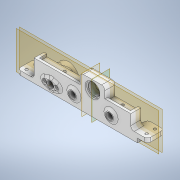
# Autodesk Inventor part: MotorBracket_v6.2
Saved by Autodesk Inventor 2022 (Build 260153000, 153)
## iProperties
Created: 2022-01-31
Part Number: MotorBracket_v6.2
Material: ABS プラスチック
Document SubType Name: Modeling
Designer: shiokaze
Density: 1.06 g/cm^3
Appearance: 滑らか - 白
Mass: 5.74152 g
Surface Area: 41.0545 cm^2
Volume: 5.41653 cm^3
Author: shiokaze
Autodesk Inventor part; units mm, degrees
ref_plane "YZ Plane" through (0, 0, 0) normal (1, 0, 0) x (0, 1, 0)
ref_plane "XZ Plane" through (0, 0, 0) normal (0, 1, 0) x (-1, 0, 0)
ref_plane "XY Plane" through (0, 0, 0) normal (0, 0, 1) x (1, 0, 0)
sketch "スケッチ2" plane through (0, 0, 0) normal (0, 0, 1) x (1, 0, 0)
  line L0 (-46.5, 9.7) -> (31.5, 9.7)
  line L1 (31.5, 9.7) -> (31.5, -9.7)
  line L2 (31.5, -9.7) -> (-46.5, -9.7)
  line L3 (-46.5, -9.7) -> (-46.5, 9.7)
  line L4 (-46.5, 9.7) -> (31.5, -9.7)
  line L5 (31.5, 9.7) -> (-46.5, -9.7)
  line L6 (-46.5, 9.7) -> (-8.95, 9.7)
  line L7 (-8.95, 9.7) -> (-8.95, -7.2)
  line L8 (-8.95, -7.2) -> (-46.5, -7.2)
  line L9 (-46.5, -7.2) -> (-46.5, 9.7)
  line L10 (31.5, 9.7) -> (5.95, 9.7)
  line L11 (5.95, 9.7) -> (5.95, -4.7)
  line L12 (5.95, -4.7) -> (31.5, -4.7)
  line L13 (31.5, -4.7) -> (31.5, 9.7)
  line L14 (-36.448454, -7.2) -> (-36.5, -7.2)
  line L15 (-36.5, -7.2) -> (-36.5, 3.5)
  line L16 (-36.5, 3.5) -> (-8.95, 3.5)
  line L17 (-8.95, 3.5) -> (-8.95, -0.360641)
  line L18 (5.95, -4.7) -> (21.5, -4.7)
  line L19 (21.5, -4.7) -> (21.5, 3.5)
  line L20 (21.5, 3.5) -> (5.95, 3.5)
  line L21 (5.95, 3.5) -> (5.95, -4.7)
  line L22 (31.5, -9.7) -> (25.5, -9.7)
  line L23 (25.5, -9.7) -> (25.5, -7.2)
  line L24 (25.5, -7.2) -> (31.5, -7.2)
  line L25 (31.5, -7.2) -> (31.5, -9.7)
  line L26 (-7.5, 0) -> (0, 0)
  point P0 (-7.5, 0)
  point P1 (5.95, 9.7)
  point P2 (-8.95, 9.7)
  point P3 (-8.95, 3.5)
  point P4 (-36.5, -7.2)
  point P5 (-46.5, -7.2)
  point P6 (31.5, -7.2)
  point P7 (31.5, -4.7)
  point P8 (21.5, -4.7)
  dimension "d0" = 78
  dimension "d1" = 19.4
  dimension "d15" = 37.55
  dimension "d16" = 2.5
  dimension "d17" = 25.55
  dimension "d18" = 6
  dimension "d19" = 2.5
  dimension "d20" = 10
  dimension "d21" = 10
  dimension "d26" = 7.5
  dimension "d188" = 10.7
  dimension "d241" = 5
  constraints: 54 end point, 12 parallel, 7 horizontal, 6 perpendicular, 3 collinear, 2 midpoint, 2 point on line, 1 coincident
  measures "d0" distance of L0.start L0.end
  measures "d1" distance of L0.end L1.end
  measures "d15" distance of L7.end L8.end
  measures "d16" distance between parallel lines of L2 L8
  measures "d17" distance of L12.end L11.end
  measures "d18" distance of L23.end L24.end
  measures "d19" distance of L22.end L23.end
  measures "d20" distance between parallel lines of L1 L19
  measures "d21" distance between parallel lines of L3 L15
  measures "d26" distance of L26.start L26.end
  measures "d188" distance between parallel lines of L16 L8
  measures "d241" distance between parallel lines of L18 L2
extrude "押し出し1" add sketch "スケッチ2" along normal blind 6 contours L0 L11 L5 L4 L7 | L8 L5 L3 | L16 L7 L4 | L4 L7 L5 L8 L15 L16 | L5 L8 L7 L4 L11 L12 L23 L2 | L4 L5 L7 | L20 L5 L11 | L5 L7 L8 | L5 L11 L4 | L1 L24 L23 L4 L12 | L20 L19 L12 L4 L11 L5 | L4 L12 L11
sketch "スケッチ8" plane through (0, 0, 6) normal (0, 0, 1) x (1, 0, 0)
  circle A0 centre (-1.5, 4.258894) radius 3.8 construction
  circle A1 centre (9.625, -3.3) radius 9.65 construction
  circle A2 centre (-12.625, -3.3) radius 9.65 construction
  circle A3 centre (-26.001939, -4.7) radius 3.8 construction
  line L0 (-46.5, -9.7) -> (25.5, -9.7) construction
  circle A4 centre (-12.625, -3.3) radius 10.5
  circle A5 centre (9.625, -3.3) radius 10.5
  line L1 (-2.125, -3.3) -> (-0.875, -3.3)
  line L2 (-12.625, -3.3) -> (-1.5, 4.258894) construction
  line L3 (-1.5, 4.258894) -> (9.625, -3.3) construction
  line L4 (-26.001939, -4.7) -> (-12.625, -3.3) construction
  line L5 (-46.5, -9.7) -> (25.5, -9.7)
  line L6 (-46.5, -9.7) -> (25.5, -9.7)
  line L7 (25.5, -9.7) -> (25.5, -11.3)
  line L8 (25.5, -11.3) -> (-46.5, -11.3) construction
  line L9 (-46.5, -11.3) -> (-46.5, -9.7)
  line L10 (-46.5, -11.3) -> (25.5, -11.3)
  line L11 (25.5, -11.3) -> (25.5, -13.8)
  line L12 (25.5, -13.8) -> (-46.5, -13.8) construction
  line L13 (-46.5, -13.8) -> (-46.5, -11.3)
  line L14 (25.5, -9.7) -> (25.5, -7.2)
  line L15 (5.95, 9.7) -> (-8.95, 9.7)
  circle A6 centre (-26.001939, -4.7) radius 5
  point P0 (0, 0)
  point P1 (-1.5, 9.7)
  dimension "d123" = 21
  dimension "d124" = 21
  dimension "d29" = 7.6
  dimension "d30" = 19.3
  dimension "d31" = 19.3
  dimension "d32" = 7.6
  dimension "d132" = 1.25
  dimension "d147" = 1.6
  dimension "d148" = 2.5
  dimension "d164" = 10
  constraints: 24 end point, 7 coincident, 5 centre point, 4 horizontal, 4 parallel, 2 collinear, 2 equal length, 2 horizontal alignment, 2 perpendicular, 2 point on line, 2 tangent, 1 midpoint, 1 vertical alignment, 4 other
  measures "d29" diameter of A0
  measures "d30" diameter of A2
  measures "d31" diameter of A1
  measures "d32" diameter of A3
  measures "d132" distance of L1.start L1.end
  measures "d147" distance of L6.end L7.end
  measures "d148" distance of L10.end L11.end
  measures "d164" diameter of A6
hole "穴1" at (-12.625, -3.3, 6) at (9.625, -3.3, 6) at (-1.5, 4.258894, 6) at (-26.001939, -4.7, 6) direction (0, 0, -1) diameter 0.1 end through all
sketch "スケッチ22" plane through (0, 0, 6) normal (0, 0, 1) x (1, 0, 0)
  circle A0 centre (9.625, -3.3) radius 0.05
  circle A1 centre (-12.625, -3.3) radius 0.05
  circle A2 centre (-26.001939, -4.7) radius 0.05
  point P0 (0, 0)
  constraints: 3 coincident
hole "穴8" at (-12.625, -3.3, 6) at (9.625, -3.3, 6) direction (0, 0, -1) diameter 4 end through all
sketch "スケッチ23" plane through (0, 0, 6) normal (0, 0, 1) x (1, 0, 0)
  circle A0 centre (-1.5, 4.258894) radius 0.05
  point P0 (0, 0)
  constraints: 1 coincident
hole "穴9" at (-1.5, 4.258894, 6) direction (0, 0, -1) diameter 7 end through all
sketch "スケッチ27" plane through (0, 0, 6) normal (0, 0, 1) x (1, 0, 0)
  circle A0 centre (-26.001939, -4.7) radius 0.05
  point P0 (0, 0)
  constraints: 1 coincident
hole "穴10" at (-26.001939, -4.7, 6) direction (0, 0, -1) diameter 10.1 end through all
sketch "スケッチ28" plane through (0, 0, 6) normal (0, 0, 1) x (1, 0, 0)
  circle A0 centre (-26.001939, -4.7) radius 2
  arc A1 (-25.293067, -9.7) -> (-26.710811, -9.7) centre (-26.001939, -4.7) ccw
  arc A2 (-25.293067, -9.7) -> (-26.710811, -9.7) centre (-26.001939, -4.7) ccw
  line L0 (-25.293067, -9.7) -> (-26.710811, -9.7)
  point P0 (0, 0)
  dimension "d173" = 4
  constraints: 2 end point, 1 centre point, 1 coincident, 1 horizontal, 1 point on circle
  measures "d173" diameter of A0
extrude "押し出し8" add sketch "スケッチ28" against normal blind 1.5
sketch "スケッチ29" plane through (-26.001939, -4.7, 4.5) normal (0, 0, -1) x (1, 0, 0)
  circle A0 centre (0, 0) radius 2 projected
  point P0 (26.001939, -4.7)
  point P1 (-3.5, 0)
  point P2 (0, 3.5)
  point P3 (3.5, 0)
  point P4 (0, -3.5)
  dimension "d176" = 3.5
  dimension "d179" = 360
  constraints: 1 coincident, 1 horizontal alignment, 5 other
  measures "d176" distance of point (0, 0) point (-3.5, 0)
hole "穴11" at (-29.501939, -4.7, 4.5) at (-26.001939, -4.7, 4.5) at (-22.501939, -4.7, 4.5) direction (0, 0, 1) diameter 1.8 end through all
sketch "スケッチ30" plane through (0, 0, 0) normal (0, 0, -1) x (-1, 0, 0)
  circle A0 centre (1.5, 4.258894) radius 3.5
  circle A1 centre (1.5, 4.258894) radius 4.5
  point P0 (0, 0)
  dimension "d189" = 9
  constraints: 1 centre point, 1 coincident
  measures "d189" diameter of A1
extrude "押し出し9" cut sketch "スケッチ30" against normal blind 1
sketch "スケッチ31" plane through (-46.5, -9.7, 6) normal (0, -1, 0) x (1, 0, 0)
  line L0 (49.5, -7.5) -> (40.5, -7.5)
  line L1 (40.5, -7.5) -> (40.5, -2.5)
  line L2 (40.5, -2.5) -> (49.5, -2.5)
  line L3 (49.5, -2.5) -> (49.5, -7.5)
  line L4 (49.5, -6) -> (40.5, -6)
  line L5 (49.5, -5) -> (40.5, -5)
  line L6 (49.5, -6) -> (40.5, -6)
  line L7 (0, 0) -> (72, 0)
  line L8 (55, -1.636919) -> (35, -1.636919)
  line L9 (35, -1.636919) -> (35, -10)
  line L10 (35, -10) -> (55, -10)
  line L11 (55, -10) -> (55, -1.636919)
  point P0 (46.5, -6)
  point P1 (45, -10)
  point P2 (45, -7.5)
  dimension "d192" = 5
  dimension "d193" = 7.5
  dimension "d194" = 10
  dimension "d195" = 20
  constraints: 16 end point, 4 midpoint, 4 parallel, 2 horizontal, 2 perpendicular, 1 vertical alignment
  measures "d192" distance between parallel lines of L0 L2
  measures "d193" distance between parallel lines of L0 L7
  measures "d194" distance between parallel lines of L10 L7
  measures "d195" distance of L9.end L10.end
extrude "押し出し10" add sketch "スケッチ31" against normal blind 1.5
sketch "スケッチ32" plane through (-46.5, -9.7, 6) normal (0, -1, 0) x (1, 0, 0)
  line L0 (52.5, -7.5) -> (37.5, -7.5)
  line L1 (52.5, -7.5) -> (37.5, -7.5)
  line L2 (37.5, -7.5) -> (37.5, -2.5)
  line L3 (37.5, -2.5) -> (52.5, -2.5)
  line L4 (52.5, -2.5) -> (52.5, -7.5)
  line L5 (37.5, -7.5) -> (37.5, -6)
  line L6 (41.5, -5) -> (48.5, -5) projected
  line L7 (0, 0) -> (72, 0) projected
  point P0 (45, -2.5)
  point P1 (45, -5)
  dimension "d198" = 5
  dimension "d204" = 15
  dimension "d205" = 2.5
  constraints: 12 end point, 2 midpoint, 2 parallel, 1 collinear, 1 horizontal, 1 perpendicular, 1 vertical alignment
  measures "d198" distance of L1.end L2.end
  measures "d204" distance between parallel lines of L4 L2
  measures "d205" distance between parallel lines of L3 L7
extrude "押し出し11" add sketch "スケッチ32" along normal blind 1.6
sketch "スケッチ33" plane through (-46.5, -9.7, 6) normal (0, 1, 0) x (1, 0, 0)
  line L0 (52.5, 2.5) -> (37.5, 2.5) projected
  line L1 (37.5, 2.5) -> (37.5, 7.5) projected
  line L2 (37.5, 7.5) -> (52.5, 7.5) projected
  line L3 (52.5, 7.5) -> (52.5, 2.5) projected
extrude "押し出し12" add sketch "スケッチ33" along normal up to surface (1.5 mm away)
fillet "フィレット14" radius 2 4 edges at (6, -10.5, -1.5) (6, -10.5, 3.5) (-9, -10.5, -1.5) (-9, -10.5, 3.5)
sketch "スケッチ34" plane through (0, 0, 0) normal (0, 0, -1) x (-1, 0, 0)
  line L0 (-31.5, -4.7) -> (-21.5, -4.7)
  line L1 (-31.5, -7.2) -> (-31.5, -4.7)
  line L2 (-25.5, -7.2) -> (-31.5, -7.2)
  line L3 (-8.5, -9.7) -> (-25.5, -9.7)
  line L4 (-25.5, -9.7) -> (-25.5, -7.2)
  line L5 (-21.5, -4.7) -> (-21.5, 3.5)
  line L6 (36.5, -7.2) -> (46.5, -7.2)
  line L7 (36.5, 3.5) -> (36.5, -7.2)
  line L8 (46.5, -9.7) -> (26.710811, -9.7)
  line L9 (46.5, -7.2) -> (46.5, -9.7)
  line L10 (-31.5, -4.7) -> (-21.5, -4.7)
  line L11 (-21.5, -4.7) -> (-21.5, -7.2)
  line L12 (-21.5, -7.2) -> (-31.5, -7.2)
  line L13 (-31.5, -7.2) -> (-31.5, -4.7)
  line L14 (46.5, -9.7) -> (-25.5, -9.7)
  line L15 (-21.5, -9.7) -> (-25.5, -9.7)
  line L16 (-25.5, -9.7) -> (-25.5, -7.2)
  line L17 (-25.5, -7.2) -> (-21.5, -7.2)
  line L18 (-21.5, -7.2) -> (-21.5, -9.7)
  line L19 (36.5, -7.2) -> (46.5, -7.2)
  line L20 (46.5, -7.2) -> (46.5, -9.7)
  line L21 (46.5, -9.7) -> (36.5, -9.7)
  line L22 (36.5, -9.7) -> (36.5, -7.2)
  point P0 (0, 0)
  point P1 (26.001939, -9.7)
  point P2 (36.5, -9.7)
  point P3 (-21.5, -9.7)
  constraints: 24 end point, 6 parallel, 3 horizontal, 3 perpendicular, 2 collinear, 2 point on line
extrude "押し出し13" add sketch "スケッチ34" along normal blind 10 from surface at -6
fillet "フィレット15" radius 2 8 edges at (21.5, -7.2, -4) (21.5, -7.2, 0) (-36.5, -8.45, 0) (-36.5, -8.45, -4) (31.5, -5.95, -4) (31.5, -5.95, 6) (-46.5, -8.45, -4) (-46.5, -8.45, 6)
fillet "フィレット16" radius 2 2 edges at (21.5, -4.7, 3) (-36.5, -7.2, 3)
fillet "フィレット17" radius 1.5 5 edges at (8.5, -8.95, -4) (-11.5, -8.95, -4) (-1.5, -8.2, 0) (8.5, -8.95, 0) (-11.5, -8.95, 0)
sketch "スケッチ35" plane through (-36.5, 3.5, 0) normal (0, 1, 0) x (1, 0, 0)
  line L0 (27.55, 0) -> (0, 0) projected
  line L1 (0, 0) -> (0, -6) projected
  line L2 (27.55, -6) -> (0, -6) projected
  line L3 (27.55, 0) -> (27.55, -6) projected
  line L4 (58, 0) -> (42.45, 0) projected
  line L5 (42.45, 0) -> (42.45, -6) projected
  line L6 (58, -6) -> (42.45, -6) projected
  line L7 (58, 0) -> (58, -6) projected
  line L8 (27.55, 0) -> (1.65, 0)
  line L9 (1.65, 0) -> (1.65, -4.5)
  line L10 (1.65, -4.5) -> (27.55, -4.5)
  line L11 (27.55, -4.5) -> (27.55, 0)
  line L12 (42.45, 0) -> (56.35, 0)
  line L13 (56.35, 0) -> (56.35, -4.5)
  line L14 (56.35, -4.5) -> (42.45, -4.5)
  line L15 (42.45, -4.5) -> (42.45, 0)
  point P0 (36.5, 0)
  point P1 (1.65, 0)
  point P2 (56.35, 0)
  dimension "d211" = 25.9
  dimension "d212" = 4.5
  dimension "d215" = 13.9
  dimension "d216" = 4.5
  constraints: 16 end point, 4 parallel, 2 horizontal, 2 perpendicular, 1 coincident
  measures "d211" distance of L10.end L9.end
  measures "d212" distance of L8.end L9.end
  measures "d215" distance of L13.end L14.end
  measures "d216" distance of L12.end L13.end
extrude "押し出し14" cut sketch "スケッチ35" against normal blind 1.6 contours L3 L10 L9 L0 | L13 L14 L5 L4
sketch "スケッチ37" plane through (-36.5, 1.9, 0) normal (0, 1, 0) x (1, 0, 0)
  line L0 (27.55, 0) -> (27.55, -6) projected
  line L1 (1.65, 0) -> (27.55, 0) projected
  line L2 (42.45, 0) -> (42.45, -6) projected
  line L3 (56.35, 0) -> (56.35, -4.5) projected
  line L4 (1.65, -4.5) -> (1.65, 0) projected
  point P0 (36.5, 0)
  point P1 (14.6, -2.25)
  point P2 (49.4, -2.25)
  dimension "d220" = 2.25
  dimension "d264" = 6.95
  dimension "d265" = 12.95
  constraints: 1 horizontal alignment
  measures "d220" distance from line of L1 point (14.6, -2.25)
  measures "d264" distance from line of L3 point (49.4, -2.25)
  measures "d265" distance from line of L4 point (14.6, -2.25)
hole "穴12" at (-21.9, 1.9, 2.25) at (12.9, 1.9, 2.25) direction (0, -1, 0) diameter 1.567 depth 0.1 tip angle 118 thread size "M2x0.4" class "6H" standard "ISO Metric profile"
ref_plane "作業平面3" through (-7.5, -7.2, 4) normal (1, 0, 0) x (0, 0, -1)
ref_plane "作業平面4" through (-1.5, 3.5, 6) normal (-1, 0, 0) x (0, 0, 1)
ref_plane "作業平面5" through (-7, -9.7, 1) normal (0, 0, 1) x (1, 0, 0)
ref_plane "作業平面6" through (0, 0, 3) normal (0, 0, 1) x (1, 0, 0)
sketch "スケッチ40" plane through (23.5, -4.7, -4) normal (0, 1, 0) x (1, 0, 0)
  line L0 (8, -10) -> (5, -10)
  line L1 (5, -10) -> (5, -7.5)
  line L2 (5, -7.5) -> (8, -7.5)
  line L3 (8, -7.5) -> (8, -10)
  line L4 (6, -10) -> (0, -10) projected
  line L5 (8, -2) -> (8, -8) projected
  point P0 (-23.5, -4)
  dimension "d231" = 3
  dimension "d232" = 2.5
  constraints: 8 end point, 2 collinear, 2 parallel, 1 coincident, 1 horizontal, 1 perpendicular
  measures "d231" distance of L1.end L2.end
  measures "d232" distance of L0.end L1.end
hole "穴13" at (28.5, -4.7, 3.5) direction (0, -1, 0) diameter 1.567 depth 0.1 tip angle 118 thread size "M2x0.4" class "6H" standard "ISO Metric profile"
mirror "ミラー2" about plane through (-7, -9.7, 1) normal (0, 0, 1) of "穴13"
fillet "フィレット18" radius 2 2 edges at (5.95, 9.7, 3) (-8.95, 9.7, 3)
sketch "スケッチ42" plane through (-44.5, -7.2, -4) normal (0, 1, 0) x (1, 0, 0)
  line L0 (6, -10) -> (0, -10) projected
  line L1 (-2, -2) -> (-2, -8) projected
  line L2 (-2, -10) -> (1, -10)
  line L3 (1, -10) -> (1, -7.5)
  line L4 (1, -7.5) -> (-2, -7.5)
  line L5 (-2, -7.5) -> (-2, -10)
  point P0 (44.5, -4)
  dimension "d242" = 3
  dimension "d243" = 2.5
  constraints: 8 end point, 2 parallel, 1 coincident, 1 collinear, 1 horizontal, 1 perpendicular, 1 point on line
  measures "d242" distance of L4.end L3.end
  measures "d243" distance of L3.end L2.end
hole "穴14" at (-43.5, -7.2, 3.5) direction (0, -1, 0) diameter 1.567 depth 0.1 tip angle 118 thread size "M2x0.4" class "6H" standard "ISO Metric profile"
mirror "ミラー4" about plane through (-7, -9.7, 1) normal (0, 0, 1) of "穴14"
sketch "スケッチ43" plane through (0, 0, 6) normal (0, 0, 1) x (1, 0, 0)
  circle A0 centre (9.625, -3.3) radius 2 projected
  circle A1 centre (9.625, -3.3) radius 2.5
  circle A2 centre (-12.625, -3.3) radius 2 projected
  circle A3 centre (-12.625, -3.3) radius 2.5
  point P0 (0, 0)
  dimension "d251" = 5
  dimension "d252" = 5
  constraints: 2 centre point, 2 coincident
  measures "d251" diameter of A1
  measures "d252" diameter of A3
extrude "押し出し15" add sketch "スケッチ43" along normal blind 1
fillet "フィレット19" radius 2 2 edges at (7.125, -3.3, 6) (-15.125, -3.3, 6)
sketch "スケッチ44" plane through (0, 0, 6) normal (0, 0, 1) x (1, 0, 0)
  circle A0 centre (-1.5, 4.258894) radius 4.5
  point P0 (0, 0)
extrude "押し出し16" cut sketch "スケッチ44" against normal blind 1
chamfer "面取り1" distance 0.2 angle 45 2 edges at (-1.5, 7.7589, 1) (-1.5, 7.7589, 5)
sketch "スケッチ45" plane through (0, 0, 0) normal (0, 0, -1) x (-1, 0, 0)
  arc A0 (26.710811, -9.7) -> (25.293067, -9.7) centre (26.001939, -4.7) ccw
  arc A1 (30.310071, -9.7) -> (21.693807, -9.7) centre (26.001939, -4.7) ccw
  line L0 (44.5, -9.7) -> (-25.5, -9.7)
  line L1 (25.293067, -9.7) -> (13, -9.7)
  line L2 (34.85, 1.9) -> (8.95, 1.9)
  line L3 (34.5, -9.7) -> (13, -9.7)
  point P0 (0, 0)
  point P1 (26.001939, -9.7)
  point P2 (21.693807, -9.7)
  point P3 (30.310071, -9.7)
  point P4 (26.710811, -9.7)
  constraints: 2 point on circle, 2 point on line, 1 centre point, 1 coincident, 1 tangent, 1 other
extrude "押し出し17" add sketch "スケッチ45" along normal up to surface (4 mm away) contours A0 L0 A1
fillet "フィレット20" radius 2 2 edges at (-19.8149, -2.4022, 0) (-32.189, -2.4022, 0)
sketch "スケッチ46" plane through (0, 0, 6) normal (0, 0, 1) x (1, 0, 0)
  circle A0 centre (-29.501939, -4.7) radius 0.9
  circle A1 centre (-26.001939, -4.7) radius 2
  circle A2 centre (-22.501939, -4.7) radius 0.9
  circle A3 centre (-29.501939, -4.7) radius 1.4
  circle A4 centre (-26.001939, -4.7) radius 2.5
  circle A5 centre (-22.501939, -4.7) radius 1.4
  line L0 (-29.941939, -6.02906) -> (-26.787653, -7.073321)
  line L1 (-25.216225, -7.073321) -> (-22.061939, -6.02906)
  line L2 (-29.941939, -3.37094) -> (-26.787653, -2.326679)
  line L3 (-25.216225, -2.326679) -> (-22.061939, -3.37094)
  point P0 (0, 0)
  point P1 (-28.364796, -3.883357)
  point P2 (-28.364796, -5.516643)
  point P3 (-23.639082, -5.516643)
  point P4 (-23.639082, -3.883357)
  dimension "d266" = 0.5
  dimension "d267" = 0.5
  dimension "d268" = 0.5
  constraints: 8 end point, 8 point on circle, 8 tangent, 3 centre point
  measures "d266" radial gap between concentric circles of A0 A3
  measures "d267" radial gap between concentric circles of A1 A4
  measures "d268" radial gap between concentric circles of A2 A5
extrude "押し出し18" add sketch "スケッチ46" along normal blind 0.9
fillet "フィレット21" radius 2 8 edges at (-30.9019, -4.7, 6) (-28.3648, -2.8488, 6) (-26.0019, -2.2, 6) (-23.6391, -2.8488, 6) (-21.1019, -4.7, 6) (-23.6391, -6.5512, 6) (-26.0019, -7.2, 6) (-28.3648, -6.5512, 6)
chamfer "面取り2" distance 0.5 angle 45 2 edges at (-30.4019, -4.7, 6.9) (-23.4019, -4.7, 6.9)
sketch "スケッチ48" plane through (0, 0, 0) normal (0, 0, -1) x (-1, 0, 0)
  line L0 (-3.207135, -2.282379) -> (6.83595, -2.282379) construction
  line L1 (6.83595, -2.282379) -> (6.83595, -5.45882) construction
  line L2 (6.83595, -5.45882) -> (-3.207135, -5.45882) construction
  line L3 (-3.207135, -5.45882) -> (-3.207135, -2.282379) construction
  line L4 (-1.132322, -3.107364) -> (-1.994358, -5.394599)
  line L5 (-1.994358, -5.394599) -> (-2.34016, -5.394599)
  line L6 (-2.34016, -5.394599) -> (-3.194785, -3.107364)
  line L7 (-3.194785, -3.107364) -> (-2.777353, -3.107364)
  line L8 (-2.777353, -3.107364) -> (-2.152439, -4.868486)
  line L9 (-2.152439, -4.868486) -> (-1.532464, -3.107364)
  line L10 (-1.532464, -3.107364) -> (-1.132322, -3.107364)
  spline S0 degree 2 poles (1.028942, -4.406593) (1.028942, -4.641244) (0.873331, -5.038917) (0.74242, -5.172298) knots 0 0 0 1 2 2 2
  spline S1 degree 2 poles (0.74242, -5.172298) (0.60657, -5.313089) (0.265707, -5.45882) (0.060696, -5.45882) knots 0 0 0 1 2 2 2
  spline S2 degree 2 poles (0.060696, -5.45882) (-0.144315, -5.45882) (-0.482708, -5.320499) (-0.611148, -5.182178) knots 0 0 0 1 2 2 2
  spline S3 degree 2 poles (-0.611148, -5.182178) (-0.769229, -5.016687) (-0.947071, -4.460933) (-0.947071, -4.05585) knots 0 0 0 1 2 2 2
  spline S4 degree 2 poles (-0.947071, -4.05585) (-0.947071, -3.658178) (-0.78405, -3.018444) (-0.613618, -2.781322) knots 0 0 0 1 2 2 2
  spline S5 degree 2 poles (-0.613618, -2.781322) (-0.448127, -2.54914) (0.075516, -2.289789) (0.418848, -2.289789) knots 0 0 0 1 2 2 2
  spline S6 degree 2 poles (0.418848, -2.289789) (0.520119, -2.289789) (0.69796, -2.309549) (0.764651, -2.331779) knots 0 0 0 1 2 2 2
  line L11 (0.764651, -2.331779) -> (0.764651, -2.724512)
  line L12 (0.764651, -2.724512) -> (0.74736, -2.724512)
  spline S7 degree 2 poles (0.74736, -2.724512) (0.69055, -2.694871) (0.483069, -2.643001) (0.364508, -2.643001) knots 0 0 0 1 2 2 2
  spline S8 degree 2 poles (0.364508, -2.643001) (-0.015875, -2.643001) (-0.482708, -3.156764) (-0.527168, -3.660648) knots 0 0 0 1 2 2 2
  spline S9 degree 2 poles (-0.527168, -3.660648) (-0.381437, -3.559377) (-0.075155, -3.448226) (0.107626, -3.448226) knots 0 0 0 1 2 2 2
  spline S10 degree 2 poles (0.107626, -3.448226) (0.285467, -3.448226) (0.552229, -3.519857) (0.69796, -3.628538) knots 0 0 0 1 2 2 2
  spline S11 degree 2 poles (0.69796, -3.628538) (0.865921, -3.754508) (1.028942, -4.144771) (1.028942, -4.406593) knots 0 0 0 1 2 2 2
  spline S12 degree 2 poles (0.61398, -4.423883) (0.61398, -4.236162) (0.515179, -3.98175) (0.406498, -3.892829) knots 0 0 0 1 2 2 2
  spline S13 degree 2 poles (0.406498, -3.892829) (0.324988, -3.828609) (0.122446, -3.786619) (0.016236, -3.786619) knots 0 0 0 1 2 2 2
  spline S14 degree 2 poles (0.016236, -3.786619) (-0.127025, -3.786619) (-0.396257, -3.873069) (-0.527168, -3.95458) knots 0 0 0 1 2 2 2
  spline S15 degree 2 poles (-0.527168, -3.95458) (-0.529638, -3.99904) (-0.534578, -4.083021) (-0.534578, -4.147241) knots 0 0 0 1 2 2 2
  spline S16 degree 2 poles (-0.534578, -4.147241) (-0.534578, -4.463403) (-0.411077, -4.851196) (-0.317217, -4.952466) knots 0 0 0 1 2 2 2
  spline S17 degree 2 poles (-0.317217, -4.952466) (-0.230766, -5.048797) (-0.043045, -5.125367) (0.063166, -5.125367) knots 0 0 0 1 2 2 2
  spline S18 degree 2 poles (0.063166, -5.125367) (0.310168, -5.125367) (0.61398, -4.774625) (0.61398, -4.423883) knots 0 0 0 1 2 2 2
  line L13 (2.044119, -5.394599) -> (1.555056, -5.394599)
  line L14 (1.555056, -5.394599) -> (1.555056, -4.811675)
  line L15 (1.555056, -4.811675) -> (2.044119, -4.811675)
  line L16 (2.044119, -4.811675) -> (2.044119, -5.394599)
  line L17 (4.538835, -5.394599) -> (2.659153, -5.394599)
  line L18 (2.659153, -5.394599) -> (2.659153, -4.962346)
  spline S19 degree 2 poles (2.659153, -4.962346) (2.861694, -4.772155) (3.222317, -4.418943) (3.395218, -4.228751) knots 0 0 0 1 2 2 2
  spline S20 degree 2 poles (3.395218, -4.228751) (3.74349, -3.845899) (3.997902, -3.386476) (3.997902, -3.141944) knots 0 0 0 1 2 2 2
  spline S21 degree 2 poles (3.997902, -3.141944) (3.997902, -3.013504) (3.918861, -2.820842) (3.847231, -2.759092) knots 0 0 0 1 2 2 2
  spline S22 degree 2 poles (3.847231, -2.759092) (3.7756, -2.697341) (3.587879, -2.635591) (3.474258, -2.635591) knots 0 0 0 1 2 2 2
  spline S23 degree 2 poles (3.474258, -2.635591) (3.365578, -2.635591) (3.143276, -2.689931) (3.042006, -2.731922) knots 0 0 0 1 2 2 2
  spline S24 degree 2 poles (3.042006, -2.731922) (2.955555, -2.766502) (2.795004, -2.865303) (2.745604, -2.899883) knots 0 0 0 1 2 2 2
  line L19 (2.745604, -2.899883) -> (2.723373, -2.899883)
  line L20 (2.723373, -2.899883) -> (2.723373, -2.46516)
  spline S25 degree 2 poles (2.723373, -2.46516) (2.849344, -2.403409) (3.301357, -2.282379) (3.503899, -2.282379) knots 0 0 0 1 2 2 2
  spline S26 degree 2 poles (3.503899, -2.282379) (3.931211, -2.282379) (4.412865, -2.734392) (4.412865, -3.119714) knots 0 0 0 1 2 2 2
  spline S27 degree 2 poles (4.412865, -3.119714) (4.412865, -3.300025) (4.328884, -3.601367) (4.254784, -3.729808) knots 0 0 0 1 2 2 2
  spline S28 degree 2 poles (4.254784, -3.729808) (4.180683, -3.863189) (3.965792, -4.125011) (3.847231, -4.250982) knots 0 0 0 1 2 2 2
  spline S29 degree 2 poles (3.847231, -4.250982) (3.65457, -4.460933) (3.182797, -4.910476) (3.042006, -5.041387) knots 0 0 0 1 2 2 2
  line L21 (3.042006, -5.041387) -> (4.538835, -5.041387)
  line L22 (4.538835, -5.041387) -> (4.538835, -5.394599)
  point P0 (0, 0)
  constraints: 2 other
extrude "押し出し19" cut sketch "スケッチ48" against normal blind 0.2
